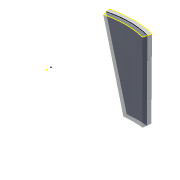
# Autodesk Inventor part: Midsurf
Saved by Autodesk Inventor 2014 (Build 180170000, 170)
## iProperties
Created: 2014-01-15
Part Number: Midsurf
Material: Generic
Document SubType Name: Modeling
Designer: Yogesh
Density: 1 g/cm^3
Appearance: Default
Author: Yogesh
Autodesk Inventor part; units mm, degrees
ref_plane "YZ Plane" through (0, 0, 0) normal (1, 0, 0) x (0, 1, 0)
ref_plane "XZ Plane" through (0, 0, 0) normal (0, 1, 0) x (-1, 0, 0)
sketch "Sketch1" plane through (0, 0, 0) normal (0, 0, 1) x (1, 0, 0)
  arc A0 (50, 0) -> (0, 0) centre (25, -96.8246) ccw
  arc A1 (52.5042, 9.6987) -> (-2.5042, 9.6987) centre (25, -96.8246) ccw
  line L0 (-2.5042, 9.6987) -> (0, 0)
  line L1 (50, 0) -> (52.5042, 9.6987)
  constraints: 5 point on circle, 4 end point, 2 centre point
ref_plane "Work Plane1" through (0, 0, -100) normal (0, 0, 1) x (1, 0, 0)
sketch "Sketch2" plane through (0, 0, -100) normal (0, 0, 1) x (1, 0, 0)
  arc A0 (50.059, 0) -> (25.7029, 0) centre (37.881, -99.2557) ccw
  arc A1 (51.2879, 10.0158) -> (24.4741, 10.0158) centre (37.881, -99.2557) ccw
  line L0 (24.4741, 10.0158) -> (25.7029, 0)
  line L1 (50.059, 0) -> (51.2879, 10.0158)
  point P0 (0, 0)
  constraints: 4 end point, 4 point on circle, 2 centre point
loft "Loft1" add profiles "Sketch1", "Sketch2"
surface_offset "OffsetSrf1"
sketch "Sketch3" plane through (25, -96.8246, 0) normal (0, 0, 1) x (1, 0, 0)
  arc A0 (25, 96.8246) -> (-25, 96.8246) centre (0, 0) ccw projected
  line L0 (25, 96.8246) -> (27.5042, 106.5233) projected
  arc A1 (27.5042, 106.5233) -> (-27.5042, 106.5233) centre (0, 0) ccw projected
  line L1 (-27.5042, 106.5233) -> (-25, 96.8246) projected
  arc A2 (26.2521, 101.6739) -> (-26.2521, 101.6739) centre (0, 5.1813) ccw
  constraints: 2 midpoint, 2 point on circle, 1 centre point
body "Solid1"
body "Srf1"
